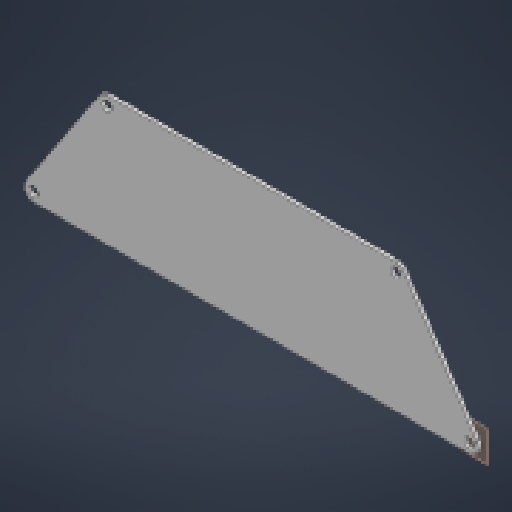
# Autodesk Inventor part: PolyRamp1
Saved by Autodesk Inventor 2026.1 (Build 301233000, 233)
## iProperties
Created: 2025-09-08
Part Number: PolyRamp1
Material: Generic
Document SubType Name: Modeling
Designer: Teddy
Density: 1 g/cm^3
Appearance: Default
Author: Teddy
Autodesk Inventor part; units mm, degrees
ref_plane "YZ Plane" through (0, 0, 0) normal (1, 0, 0) x (0, 1, 0)
ref_plane "XZ Plane" through (0, 0, 0) normal (0, 1, 0) x (-1, 0, 0)
ref_plane "XY Plane" through (0, 0, 0) normal (0, 0, 1) x (1, 0, 0)
ref_plane "Work Plane1" through (34.6079, -51.2355, 0) normal (0, 0, 1) x (1, 0, 0)
sketch "Sketch1" plane through (34.6079, -51.2355, 0) normal (0, 0, 1) x (1, 0, 0)
  circle A0 centre (-180.6291, 37.0026) radius 4.445
  circle A1 centre (-209.2228, -4.986) radius 4.445
  circle A2 centre (-31.2607, 37.0797) radius 4.445
  circle A3 centre (-2.667, -4.9089) radius 4.445
  line L0 (-180.6314, 41.4476) -> (-31.263, 41.5247)
  line L1 (-27.5867, 39.5816) -> (1.007, -2.407)
  line L2 (-2.6654, -9.3539) -> (-209.2211, -9.431)
  line L3 (-184.3031, 39.5045) -> (-212.8968, -2.484)
  circle A4 centre (-2.667, -4.9089) radius 2.286 projected
  circle A5 centre (-180.6291, 37.0026) radius 2.286 projected
  circle A6 centre (-209.2228, -4.986) radius 2.286 projected
  circle A7 centre (-31.2607, 37.0797) radius 2.286 projected
  point P0 (-34.6079, 51.2355)
  dimension "d0" = 8.89
  dimension "d1" = 8.89
  dimension "d2" = 8.89
  dimension "d3" = 8.89
  constraints: 8 end point, 8 point on circle, 8 tangent, 4 centre point, 4 coincident
  measures "d0" diameter of A0
  measures "d1" diameter of A1
  measures "d2" diameter of A2
  measures "d3" diameter of A3
extrude "Extrusion1" add sketch "Sketch1" along normal blind 1.5875
body "Solid1"
